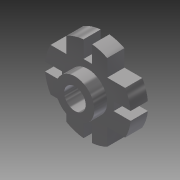
# Autodesk Inventor part: 3-3
Saved by Autodesk Inventor 2015 SP2 (Build 190223200, 223)
## iProperties
Created: 2015-09-14
Part Number: 3-3
Material: Iron, Malleable
Document SubType Name: Modeling
Designer: Brandon
Density: 7.15 g/cm^3
Appearance: Semi-Polished
Author: Brandon
Autodesk Inventor part; units mm, degrees
ref_plane "YZ Plane" through (0, 0, 0) normal (1, 0, 0) x (0, 1, 0)
ref_plane "XZ Plane" through (0, 0, 0) normal (0, 1, 0) x (-1, 0, 0)
ref_plane "XY Plane" through (0, 0, 0) normal (0, 0, 1) x (1, 0, 0)
sketch "Sketch1" plane through (0, 0, 0) normal (0, 0, 1) x (1, 0, 0)
  circle A0 centre (0, 0) radius 63.5
  dimension "d0" = 127
  constraints: 1 centre point, 1 coincident
  measures "d0" diameter of A0
extrude "Extrusion1" add sketch "Sketch1" along normal blind 25.4
sketch "Sketch2" plane through (0, 0, 25.4) normal (0, 0, 1) x (1, 0, 0)
  circle A0 centre (0, 0) radius 28.575
  dimension "d3" = 57.15
  constraints: 1 centre point, 1 coincident
  measures "d3" diameter of A0
extrude "Extrusion2" add sketch "Sketch2" along normal blind 19.05
sketch "Sketch3" plane through (0, 0, 44.45) normal (0, 0, 1) x (1, 0, 0)
  circle A0 centre (0, 0) radius 15.875
  dimension "d6" = 31.75
  constraints: 1 centre point, 1 coincident
  measures "d6" diameter of A0
extrude "Extrusion3" cut sketch "Sketch3" against normal through all
sketch "Sketch4" plane through (0, 0, 25.4) normal (0, 0, 1) x (1, 0, 0)
  line L0 (0, 0) -> (0, 38.1)
  line L1 (0, 38.1) -> (0, -38.1)
  line L2 (0, -38.1) -> (6.35, -38.1)
  line L3 (6.35, -38.1) -> (6.35, -63.1817)
  circle A0 centre (0, 0) radius 63.5 projected
  line L4 (0, -38.1) -> (-6.35, -38.1)
  line L5 (-6.35, -38.1) -> (-6.35, -80.9216)
  line L6 (-6.35, -80.9216) -> (6.35, -63.1817)
  line L7 (0, 38.1) -> (6.35, 38.1)
  line L8 (6.35, 38.1) -> (6.35, 68.5855)
  line L9 (0, 38.1) -> (-6.35, 38.1)
  line L10 (-6.35, 38.1) -> (-6.35, 68.5855)
  line L11 (-6.35, 68.5855) -> (6.35, 68.5855)
  dimension "d9" = 38.1
  dimension "d10" = 76.2
  dimension "d11" = 6.35
  dimension "d12" = 6.35
  dimension "d13" = 6.35
  dimension "d14" = 6.35
  constraints: 24 end point, 5 perpendicular, 4 horizontal, 1 point on line, 1 vertical, 2 other
  measures "d9" distance of L0.start L0.end
  measures "d10" distance of L0.end L1.end
  measures "d11" distance of L1.end L2.end
  measures "d12" distance of L1.end L4.end
  measures "d13" distance of L0.end L7.end
  measures "d14" distance of L0.end L9.end
extrude "Extrusion4" cut sketch "Sketch4" against normal through all contours L9 L10 A0 L8 L7 | L2 L3 A0 L5 L4 | A0 L10 L11 L8 | L6 L5 A0
sketch "Sketch5" plane through (0, 0, 25.4) normal (0, 0, 1) x (1, 0, 0)
  line L0 (0, 0) -> (38.1, 0)
  line L1 (38.1, 0) -> (-38.1, 0)
  line L2 (-38.1, 0) -> (-38.1, 6.35)
  line L3 (-38.1, 6.35) -> (-99.0804, 6.35)
  line L4 (-38.1, 0) -> (-38.1, -6.35)
  line L5 (-38.1, -6.35) -> (-95.4724, -6.35)
  line L6 (-95.4724, -6.35) -> (-99.0804, 6.35)
  line L7 (38.1, 0) -> (38.1, -6.35)
  line L8 (38.1, -6.35) -> (92.4195, -6.35)
  line L9 (38.1, 0) -> (38.1, 6.35)
  line L10 (38.1, 6.35) -> (95.1949, 6.35)
  line L11 (95.1949, 6.35) -> (92.4195, -6.35)
  dimension "d17" = 38.1
  dimension "d18" = 76.2
  dimension "d19" = 6.35
  dimension "d20" = 6.35
  dimension "d21" = 6.35
  dimension "d22" = 6.35
  constraints: 24 end point, 5 perpendicular, 3 vertical, 1 horizontal, 1 point on line
  measures "d17" distance of L0.start L0.end
  measures "d18" distance of L0.end L1.end
  measures "d19" distance of L1.end L2.end
  measures "d20" distance of L1.end L4.end
  measures "d21" distance of L0.end L7.end
  measures "d22" distance of L0.end L9.end
extrude "Extrusion5" cut sketch "Sketch5" against normal through all
sketch "Sketch6" plane through (0, 0, 25.4) normal (0, 0, 1) x (1, 0, 0)
  point P0 (0, 0)
sketch "Sketch7" plane through (0, 0, 25.4) normal (0, 0, 1) x (1, 0, 0)
  line L0 (0, 0) -> (31.75, 0)
  line L1 (0, 0) -> (0, 31.75)
  line L2 (0, 31.75) -> (124.8927, 31.75)
  line L3 (0, 0) -> (0, -31.75)
  line L4 (0, 0) -> (-31.75, 0)
  line L5 (-31.75, 0) -> (-145.867, 0)
  line L6 (0, 31.75) -> (-126.7995, 31.75)
  line L7 (0, -31.75) -> (-134.9032, -31.75)
  line L8 (0, -31.75) -> (128.2295, -31.75)
  line L9 (-31.75, -31.75) -> (-31.75, -121.3175)
  line L10 (-31.75, -121.3175) -> (-134.9032, -31.75)
  line L11 (28.575, -31.75) -> (28.575, -121.3175)
  line L12 (28.575, -121.3175) -> (128.2295, -31.75)
  line L13 (28.575, 31.75) -> (28.575, 107.95)
  line L14 (28.575, 107.95) -> (124.8927, 31.75)
  line L15 (-126.7995, 31.75) -> (-31.75, 99.6281)
  line L16 (-31.75, 99.6281) -> (-31.75, 31.75)
  dimension "d25" = 31.75
  dimension "d26" = 31.75
  dimension "d27" = 31.75
  dimension "d28" = 31.75
  dimension "d29" = 76.2
  constraints: 34 end point, 6 horizontal, 5 point on line, 4 vertical, 2 perpendicular
  measures "d25" distance of L0.start L0.end
  measures "d26" distance of L0.start L1.end
  measures "d27" distance of L0.start L3.end
  measures "d28" distance of L0.start L4.end
  measures "d29" distance of L13.start L13.end
extrude "Extrusion6" cut sketch "Sketch7" against normal through all
body "Solid1"
